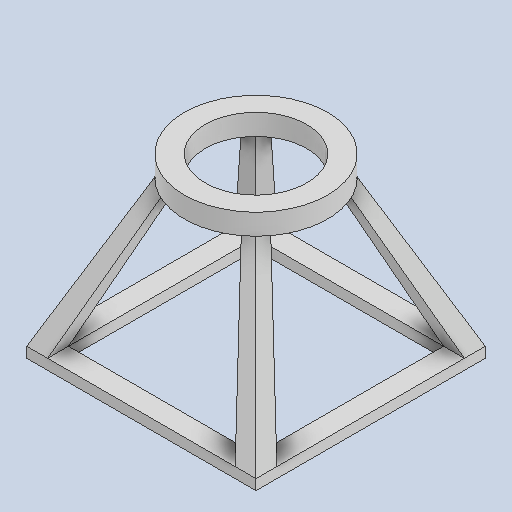
# Autodesk Inventor part: klec_1
Saved by Autodesk Inventor 2025 (Build 290162000, 162)
## iProperties
Created: 2025-04-20
Part Number: klec_1
Material: Generic
Document SubType Name: Sheet Metal
Designer: Pravoslav
Density: 1 g/cm^3
Sheet Metal Rule: Default_mm
Appearance: Default
Author: Pravoslav
Autodesk Inventor part; units mm, degrees
ref_plane "YZ Plane" through (0, 0, 0) normal (1, 0, 0) x (0, 1, 0)
ref_plane "XZ Plane" through (0, 0, 0) normal (0, 1, 0) x (-1, 0, 0)
sketch "Sketch1" plane through (0, 0, 0) normal (0, 1, 0) x (-1, 0, 0)
  circle A0 centre (0, 0) radius 24.35
  circle A1 centre (0, 0) radius 34.35
  dimension "d0" = 48.7
  dimension "d1" = 10
  constraints: 2 centre point, 2 coincident
  measures "d0" diameter of A0
  measures "d1" radial gap between concentric circles of A1 A0
extrude "Extrusion1" add sketch "Sketch1" along normal blind 10
ref_plane "Work Plane1" through (0, -70, 0) normal (0, -1, 0) x (1, 0, 0)
sketch "Sketch2" plane through (0, -70, 0) normal (0, -1, 0) x (1, 0, 0)
  circle A0 centre (0, 0) radius 34.35 projected
  circle A1 centre (0, 0) radius 24.35 projected
  line L0 (55, 55) -> (-55, 55)
  line L1 (-55, 55) -> (-55, -55)
  line L2 (-55, -55) -> (55, -55)
  line L3 (55, -55) -> (55, 55)
  line L4 (55, 55) -> (-55, -55) construction
  line L5 (-55, 55) -> (55, -55) construction
  line L6 (45, 45) -> (-45, 45)
  line L7 (-45, 45) -> (-45, -45)
  line L8 (-45, -45) -> (45, -45)
  line L9 (45, -45) -> (45, 45)
  line L10 (45, 45) -> (-45, -45) construction
  line L11 (-45, 45) -> (45, -45) construction
  dimension "d7" = 110
  dimension "d8" = 110
  dimension "d9" = 90
  dimension "d10" = 90
  constraints: 24 end point, 4 midpoint, 4 parallel, 2 horizontal, 2 perpendicular
  measures "d7" distance of L2.end L1.end
  measures "d8" distance of L1.end L0.end
  measures "d9" distance of L8.end L7.end
  measures "d10" distance of L7.end L6.end
extrude "Extrusion2" add sketch "Sketch2" along normal blind 5 contours L3 L2 L1 L0
sketch "Sketch3" plane through (0, -70, 0) normal (0, 1, 0) x (1, 0, 0)
  line L0 (-55, 55) -> (55, 55) projected
  line L1 (45, -45) -> (45, 45) projected
  line L2 (55, 55) -> (45, 55)
  line L3 (45, 55) -> (45, 45)
  line L4 (45, 45) -> (55, 45)
  line L5 (55, 45) -> (55, 55)
  line L6 (-45, 45) -> (-45, -45) projected
  line L7 (-55, 55) -> (-45, 55)
  line L8 (-45, 55) -> (-45, 45)
  line L9 (-45, 45) -> (-55, 45)
  line L10 (-55, 45) -> (-55, 55)
  line L11 (55, -55) -> (-55, -55) projected
  line L12 (-55, -55) -> (-45, -55)
  line L13 (-45, -55) -> (-45, -45)
  line L14 (-45, -45) -> (-55, -45)
  line L15 (-55, -45) -> (-55, -55)
  line L16 (55, -55) -> (45, -55)
  line L17 (45, -55) -> (45, -45)
  line L18 (45, -45) -> (55, -45)
  line L19 (55, -45) -> (55, -55)
  point P0 (0, 0)
  constraints: 32 end point, 8 parallel, 4 horizontal, 4 perpendicular, 1 point on line
sketch "Sketch4" plane through (0, 0, 0) normal (0, -1, 0) x (1, 0, 0)
  line L0 (-55, 55) -> (-55, -55) projected
  line L1 (-55, -55) -> (55, -55) projected
  line L2 (55, -55) -> (55, 55) projected
  line L3 (55, 55) -> (-55, 55) projected
  line L4 (45, 45) -> (45, -45) projected
  line L5 (45, -45) -> (-45, -45) projected
  line L6 (-45, -45) -> (-45, 45) projected
  line L7 (-45, 45) -> (45, 45) projected
  line L8 (55, 55) -> (-55, -55)
  line L9 (-55, 55) -> (55, -55)
  line L10 (55, -55) -> (45, -55)
  line L11 (45, -55) -> (45, -45)
  line L12 (45, -45) -> (55, -45)
  line L13 (55, -45) -> (55, -55)
  line L14 (24.4112, -24.4112) -> (17.4112, -24.4112)
  line L15 (17.4112, -24.4112) -> (17.4112, -17.4112)
  line L16 (17.4112, -17.4112) -> (24.4112, -17.4112)
  line L17 (24.4112, -17.4112) -> (24.4112, -24.4112)
  line L18 (24.4112, 17.4112) -> (17.4112, 17.4112)
  line L19 (17.4112, 17.4112) -> (17.4112, 24.4112)
  line L20 (17.4112, 24.4112) -> (24.4112, 24.4112)
  line L21 (24.4112, 24.4112) -> (24.4112, 17.4112)
  line L22 (-17.2122, 17.4112) -> (-24.2122, 17.4112)
  line L23 (-24.2122, 17.4112) -> (-24.2122, 24.4112)
  line L24 (-24.2122, 24.4112) -> (-17.2122, 24.4112)
  line L25 (-17.2122, 24.4112) -> (-17.2122, 17.4112)
  line L26 (-17.4112, -24.4112) -> (-24.4112, -24.4112)
  line L27 (-24.4112, -24.4112) -> (-24.4112, -17.4112)
  line L28 (-24.4112, -17.4112) -> (-17.4112, -17.4112)
  line L29 (-17.4112, -17.4112) -> (-17.4112, -24.4112)
  point P0 (0, 0)
  dimension "d13" = 7
  dimension "d14" = 7
  dimension "d15" = 7
  dimension "d16" = 7
  dimension "d17" = 7
  dimension "d18" = 7
  dimension "d19" = 7
  dimension "d20" = 7
  constraints: 44 end point, 10 parallel, 6 perpendicular, 5 horizontal, 3 point on line
  measures "d13" distance of L15.end L16.end
  measures "d14" distance of L14.end L15.end
  measures "d15" distance of L20.start L21.start
  measures "d16" distance of L18.end L20.start
  measures "d17" distance of L24.start L25.start
  measures "d18" distance of L22.end L24.start
  measures "d19" distance of L28.start L29.start
  measures "d20" distance of L26.end L28.start
loft "Loft1" add profiles "Sketch4", "Sketch3" contours L27 L28 L8 | L8 L29 L26 / L0 L8 L9 L10
pattern_circular "Circular Pattern1" count 4 over 360 about axis through (0, 0, 0) along (0, 1, 0) of "Loft1"
equation "\"BendRadius\" = Thickness"
equation "\"BendReliefWidth\" = Thickness"
equation "\"BendReliefDepth\" = 0.5 * Thickness"
equation "\"CornerReliefSize\" = 4 * Thickness"
equation "\"MinimumRemnant\" = 2 * Thickness"
equation "\"TransitionRadius\" = BendRadius"
equation "\"JacobiRadiusSize\" = BendRadius"
equation "\"GapSize\" = Thickness"
equation "\"Thickness\" = 0.5"
body "Solid1"
